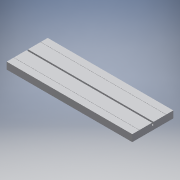
# Autodesk Inventor part: Large Bread Board
Saved by Autodesk Inventor 2018 (Build 220112000, 112)
## iProperties
Created: 2018-05-02
Part Number: Large Bread Board
Material: PC/ABS Plastic
Document SubType Name: Modeling
Designer: Ajith Thomas
Density: 0.357273 g/cm^3
Appearance: Smooth - White
Mass: 28.0506 g
Surface Area: 270.329 cm^2
Volume: 78.5131 cm^3
Author: Ajith Thomas
Autodesk Inventor part; units mm, degrees
ref_plane "YZ Plane" through (0, 0, 0) normal (1, 0, 0) x (0, 1, 0)
ref_plane "XZ Plane" through (0, 0, 0) normal (0, 1, 0) x (-1, 0, 0)
ref_plane "XY Plane" through (0, 0, 0) normal (0, 0, 1) x (1, 0, 0)
sketch "Sketch1" plane through (0, 0, 0) normal (0, 1, 0) x (-1, 0, 0)
  line L0 (82.5, -27) -> (-82.5, -27)
  line L1 (-82.5, -27) -> (-82.5, 27)
  line L2 (-82.5, 27) -> (82.5, 27)
  line L3 (82.5, 27) -> (82.5, -27)
  line L4 (82.5, -27) -> (-82.5, 27) construction
  line L5 (-82.5, -27) -> (82.5, 27) construction
  point P0 (0, 0)
  dimension "d0" = 165
  dimension "d1" = 54
  constraints: 12 end point, 2 midpoint, 2 parallel, 1 horizontal, 1 perpendicular
  measures "d0" distance of L1.end L2.end
  measures "d1" distance between parallel lines of L2 L0
extrude "Extrusion1" add sketch "Sketch1" along normal blind 9
sketch "Sketch2" plane through (82.5, 0, 27) normal (1, 0, 0) x (0, 0, -1)
  line L0 (0, 9) -> (54, 9) projected
  line L1 (27, 0) -> (27, 9) construction
  line L2 (26, 12.517) -> (28, 12.517)
  line L3 (28, 12.517) -> (28, 5.483)
  line L4 (28, 5.483) -> (26, 5.483)
  line L5 (26, 5.483) -> (26, 12.517)
  line L6 (26, 12.517) -> (28, 5.483) construction
  line L7 (28, 12.517) -> (26, 5.483) construction
  dimension "d4" = 2
  constraints: 14 end point, 3 midpoint, 2 parallel, 1 horizontal, 1 perpendicular
  measures "d4" distance of L3.end L4.end
extrude "Extrusion2" cut sketch "Sketch2" against normal blind 203.725
sketch "Sketch3" plane through (82.5, 0, 27) normal (1, 0, 0) x (0, 0, -1)
  line L0 (27, 0) -> (27, 5.483) construction
  line L1 (28, 5.483) -> (26, 5.483) construction
  line L2 (27, 2.7415) -> (44.5, 2.7415) construction
  line L3 (44.5, 2.7415) -> (44.75, 2.7415)
  line L4 (44.75, 2.7415) -> (44.75, 10.8697)
  line L5 (44.75, 10.8697) -> (44.5, 10.8697)
  line L6 (44.5, 10.8697) -> (44.5, 2.7415)
  line L7 (9.5, 2.7415) -> (9.25, 2.7415)
  line L8 (9.25, 2.7415) -> (9.25, 10.8697)
  line L9 (9.25, 10.8697) -> (9.5, 10.8697)
  line L10 (9.5, 10.8697) -> (9.5, 2.7415)
  dimension "d7" = 17.5
  dimension "d8" = 0.25
  constraints: 20 end point, 4 symmetric about line, 2 horizontal, 2 midpoint, 2 parallel, 1 perpendicular
  measures "d7" distance of L2.start L2.end
  measures "d8" distance of L5.end L4.end
extrude "Extrusion3" cut sketch "Sketch3" against normal blind 203.725
body "Solid1"
